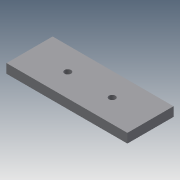
# Autodesk Inventor part: prepazka_bez_loziska
Saved by Autodesk Inventor 2013 (Build 170138000, 138)
## iProperties
Created: 2012-08-21
Part Number: prepazka_bez_loziska
Material: Generic
Document SubType Name: Modeling
Designer: idle-rug
Density: 1 g/cm^3
Author: idle-rug
Autodesk Inventor part; units mm, degrees
ref_plane "YZ Plane" through (0, 0, 0) normal (1, 0, 0) x (0, 1, 0)
ref_plane "XZ Plane" through (0, 0, 0) normal (0, 1, 0) x (-1, 0, 0)
ref_plane "XY Plane" through (0, 0, 0) normal (0, 0, 1) x (1, 0, 0)
sketch "Sketch1" plane through (0, 0, 0) normal (0, 0, 1) x (1, 0, 0)
  line L0 (65.5, 25) -> (-65.5, 25)
  line L1 (-65.5, 25) -> (-65.5, -25)
  line L2 (-65.5, -25) -> (65.5, -25)
  line L3 (65.5, -25) -> (65.5, 25)
  line L4 (65.5, 25) -> (-65.5, -25) construction
  line L5 (-65.5, 25) -> (65.5, -25) construction
  line L6 (0, 0) -> (-24.1, 0)
  line L7 (0, 0) -> (24.1, 0)
  circle A0 centre (-24.1, 0) radius 3.5
  circle A1 centre (24.1, 0) radius 3.5
  dimension "d0" = 131
  dimension "d1" = 50
  dimension "d2" = 24.1
  dimension "d3" = 24.1
  dimension "d4" = 7
  dimension "d5" = 7
  constraints: 16 end point, 3 equal length, 2 centre point, 2 coincident, 2 midpoint, 2 perpendicular, 1 horizontal
  measures "d0" distance of L2.end L1.end
  measures "d1" distance of L1.end L0.end
  measures "d2" distance of L6.start L6.end
  measures "d3" distance of L6.start L7.end
  measures "d4" diameter of A0
  measures "d5" diameter of A1
extrude "Extrusion1" add sketch "Sketch1" along normal blind 10
body "Solid1"
